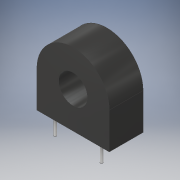
# Autodesk Inventor part: AC1015
Saved by Autodesk Inventor 2018 (Build 220112000, 112)
## iProperties
Created: 2018-03-01
Part Number: AC1015
Material: Generic
Document SubType Name: Modeling
Designer: brutu
Density: 1 g/cm^3
Appearance: Default
Author: brutu
Autodesk Inventor part; units mm, degrees
ref_plane "YZ Plane" through (0, 0, 0) normal (1, 0, 0) x (0, 1, 0)
ref_plane "XZ Plane" through (0, 0, 0) normal (0, 1, 0) x (-1, 0, 0)
ref_plane "XY Plane" through (0, 0, 0) normal (0, 0, 1) x (1, 0, 0)
sketch "Sketch1" plane through (0, 0, 0) normal (0, 0, 1) x (1, 0, 0)
  arc A0 (11.9, 11.9) -> (-11.9, 11.9) centre (0, 11.9) ccw
  line L0 (-11.9, 11.9) -> (-11.9, 0)
  line L1 (-11.9, 0) -> (11.9, 0)
  line L2 (11.9, 0) -> (11.9, 11.9)
  circle A1 centre (0, 11.9) radius 4.75
  point P0 (0, 0)
  dimension "d0" = 11.9
  dimension "d1" = 180
  dimension "d2" = 11.9
  dimension "d3" = 9.5
  dimension "d4" = 23.8
  dimension "d5" = 0
  constraints: 6 end point, 2 centre point, 2 coincident, 2 perpendicular, 2 point on circle, 1 horizontal alignment, 1 vertical, 1 vertical alignment
  measures "d0" radius of A0
  measures "d2" distance from line of L1 A0.centre
  measures "d3" diameter of A1
  measures "d4" distance of L0.end L1.end
  measures "d5" distance from line of point (0, 0) L1
extrude "Extrusion1" add sketch "Sketch1" along normal blind 1.75 and the other way blind 9.37
sketch "Sketch2" plane through (-11.9, 0, 1.75) normal (0, -1, 0) x (1, 0, 0)
  circle A0 centre (4.28, -1.75) radius 0.4065
  circle A1 centre (19.52, -1.75) radius 0.4065
  circle A2 centre (11.9, -9.37) radius 0.4065
  point P0 (11.9, -1.75)
  dimension "d10" = 0.813
  dimension "d11" = 0.813
  dimension "d12" = 15.24
  dimension "d13" = 7.62
  dimension "d14" = 0.813
  dimension "d15" = 7.62
  constraints: 3 centre point, 2 horizontal alignment, 1 vertical alignment
  measures "d10" diameter of A0
  measures "d11" diameter of A1
  measures "d12" distance of A0.centre A1.centre
  measures "d13" distance of point (11.9, -1.75) A0.centre
  measures "d14" diameter of A2
  measures "d15" distance of A2.centre point (11.9, -1.75)
extrude "Extrusion2" add sketch "Sketch2" along normal blind 6
equation "\"d11\" = d10"
equation "\"d13\" = 0.5 * d12"
equation "\"d14\" = d10"
body "Solid1"
